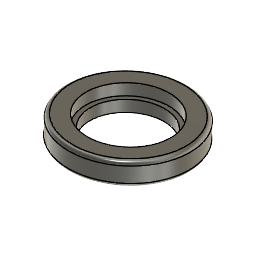
seguro clip (Autodesk Fusion 360 design; units mm, degrees)
part number: 2026-06-24-11-01-33-015
Autodesk Fusion 360 part; units mm, degrees
sketch "Boceto1" plane through (0, 0, 0) normal (1, 0, 0) x (0, 1, 0)
  circle A0 centre (0, 0) radius 8
  circle A1 centre (0, 0) radius 4.9
  dimension "d1" = 16
  dimension "d2" = 9.8
  constraint coincident A0.centre A1.centre
  measures "d1" diameter of A0
  measures "d2" diameter of A1
extrude "Extruir1" add sketch "Boceto1" against normal blind 3
move_body "Desplazar1" bodies 1 to x (0, -0.036999, -0.999315) y (0.732785, 0.679994, -0.025177) z (0.68046, -0.732283, 0.027113) at (0, 0, 0)
fillet "Empalme1" radius 0.5 1 faces at (5.2911, 6.0332, 0.7773)
sketch "Boceto3" plane through (0, 0.111, 2.9979) normal (0, 0.036999, 0.999315) x (-1, 0, 0)
  circle A0 centre (0, 0) radius 4.9
  circle A1 centre (0, 0) radius 7.5
  circle A2 centre (0, 0) radius 5.5
  dimension "d10" = 11
  constraint concentric A0 A2
  measures "d10" diameter of A2
extrude "Extruir3" cut sketch "Boceto3" against normal blind 1.5 contours A0 | A2
